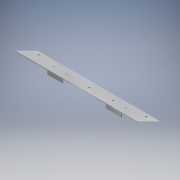
# Autodesk Inventor part: side plate
Saved by Autodesk Inventor 2016 (Build 200138000, 138)
## iProperties
Created: 2016-01-16
Part Number: side plate
Material: Aluminum 6061
Document SubType Name: Modeling
Designer: gus
Density: 2.7 g/cm^3
Appearance: Aluminum - Flat
Mass: 440.775 g
Surface Area: 1095.58 cm^2
Volume: 163.25 cm^3
User Status: complete
Author: gus
Autodesk Inventor part; units mm, degrees
ref_plane "YZ Plane" through (0, 0, 0) normal (1, 0, 0) x (0, 1, 0)
ref_plane "XZ Plane" through (0, 0, 0) normal (0, 1, 0) x (-1, 0, 0)
ref_plane "XY Plane" through (0, 0, 0) normal (0, 0, 1) x (1, 0, 0)
sketch "Sketch1" plane through (0, 0, 0) normal (0, 1, 0) x (-1, 0, 0)
  line L0 (0, 0) -> (762, 0)
  line L1 (762, 0) -> (762, 50.8)
  line L2 (762, 50.8) -> (0, 50.8)
  line L3 (0, 50.8) -> (0, 0)
  dimension "d0" = 762
  dimension "d1" = 50.8
  constraints: 8 end point, 2 parallel, 1 horizontal, 1 perpendicular
  measures "d0" distance of L2.end L1.end
  measures "d1" distance of L1.end L0.end
extrude "Extrusion1" add sketch "Sketch1" along normal blind 3.175
sketch "Sketch2" plane through (0, 3.175, 0) normal (0, 1, 0) x (1, 0, 0)
  circle A0 centre (-381, -28.575) radius 4.7625
  line L0 (0, 0) -> (-762, 0) projected
  line L1 (0, -50.8) -> (0, 0) projected
  circle A1 centre (-114.3, -12.7) radius 4.7625
  line L2 (-762, -50.8) -> (0, -50.8) projected
  circle A2 centre (-647.7, -12.7) radius 4.7625
  line L3 (-647.7, 0) -> (-647.7, -50.8) construction
  line L4 (-762, -50.8) -> (0, -50.8) construction
  line L5 (-114.3, -50.8) -> (-114.3, 0) construction
  circle A3 centre (-558.8, -25.4) radius 3.3734
  line L6 (-762, 0) -> (-762, -50.8) projected
  circle A4 centre (-495.3, -25.4) radius 3.3734
  circle A5 centre (-203.2, -25.4) radius 3.3734
  circle A6 centre (-266.7, -25.4) radius 3.3734
  dimension "d4" = 9.525
  dimension "d5" = 28.575
  dimension "d6" = 381
  dimension "d9" = 9.525
  dimension "d10" = 38.1
  dimension "d12" = 9.525
  dimension "d13" = 38.1
  dimension "d31" = 266.7
  dimension "d32" = 266.7
  dimension "d33" = 6.7469
  dimension "d34" = 203.2
  dimension "d35" = 25.4
  dimension "d36" = 6.7469
  dimension "d37" = 25.4
  dimension "d38" = 266.7
  dimension "d39" = 6.7469
  dimension "d40" = 6.7469
  dimension "d41" = 25.4
  dimension "d42" = 25.4
  dimension "d43" = 203.2
  dimension "d44" = 266.7
  constraints: 7 centre point, 6 point on line, 4 end point, 1 perpendicular, 1 vertical
  measures "d4" diameter of A0
  measures "d5" distance from line of L0 A0.centre
  measures "d6" distance from line of A0.centre L1
  measures "d9" diameter of A1
  measures "d10" distance from line of L2 A1.centre
  measures "d12" diameter of A2
  measures "d13" distance from line of L2 A2.centre
  measures "d31" distance from line of L3 A0.centre
  measures "d32" distance from line of L5 A0.centre
  measures "d33" diameter of A3
  measures "d34" distance from line of A3.centre L6
  measures "d35" distance from line of L0 A3.centre
  measures "d36" diameter of A4
  measures "d37" distance from line of L0 A4.centre
  measures "d38" distance from line of L6 A4.centre
  measures "d39" diameter of A5
  measures "d40" diameter of A6
  measures "d41" distance from line of L0 A6.centre
  measures "d42" distance from line of L0 A5.centre
  measures "d43" distance from line of L1 A5.centre
  measures "d44" distance from line of L1 A6.centre
extrude "Extrusion2" cut sketch "Sketch2" against normal blind 3.175 contours A0 | A1 | A2 | A3 | A4 | A5 | A6
sketch "Sketch3" plane through (-762, 0, 50.8) normal (0, 0, 1) x (1, 0, 0)
  line L0 (762, 3.175) -> (0, 3.175) projected
  line L1 (762, 3.175) -> (0, 3.175)
  line L2 (0, 3.175) -> (0, -19.05)
  line L3 (0, -19.05) -> (762, -19.05)
  line L4 (762, -19.05) -> (762, 3.175)
  point P0 (762, 0)
  dimension "d15" = 762
  dimension "d16" = 22.225
  constraints: 8 end point, 2 parallel, 1 horizontal, 1 perpendicular
  measures "d15" distance of L3.end L2.end
  measures "d16" distance of L2.end L1.end
extrude "Extrusion3" add sketch "Sketch3" along normal blind 3.175
sketch "Sketch4" plane through (0, 0, 0) normal (0, 0, -1) x (-1, 0, 0)
  line L0 (0, 3.175) -> (762, 3.175)
  line L1 (762, 3.175) -> (762, -19.05)
  line L2 (762, -19.05) -> (0, -19.05)
  line L3 (0, -19.05) -> (0, 3.175)
  dimension "d19" = 762
  dimension "d20" = 22.225
  constraints: 8 end point, 2 parallel, 1 horizontal, 1 perpendicular
  measures "d19" distance of L1.end L2.end
  measures "d20" distance of L0.end L1.end
extrude "Extrusion4" add sketch "Sketch4" along normal blind 3.175
sketch "Sketch5" plane through (-762, 0, 53.975) normal (0, 0, 1) x (1, 0, 0)
  line L0 (762, -19.05) -> (0, -19.05) projected
  line L1 (0, 0) -> (762, 0) projected
  line L2 (730.25, -19.05) -> (565.15, -19.05)
  line L3 (565.15, -19.05) -> (565.15, 0)
  line L4 (565.15, 0) -> (730.25, 0)
  line L5 (730.25, 0) -> (730.25, -19.05)
  line L6 (762, -19.05) -> (762, 3.175) projected
  line L7 (488.95, -19.05) -> (273.05, -19.05)
  line L8 (273.05, -19.05) -> (273.05, 0)
  line L9 (273.05, 0) -> (488.95, 0)
  line L10 (488.95, 0) -> (488.95, -19.05)
  line L11 (31.75, -19.05) -> (196.85, -19.05)
  line L12 (196.85, -19.05) -> (196.85, 0)
  line L13 (196.85, 0) -> (31.75, 0)
  line L14 (31.75, 0) -> (31.75, -19.05)
  line L15 (0, 3.175) -> (0, -19.05) projected
  dimension "d23" = 165.1
  dimension "d24" = 31.75
  dimension "d25" = 215.9
  dimension "d26" = 76.2
  dimension "d27" = 165.1
  dimension "d28" = 31.75
  constraints: 24 end point, 6 parallel, 6 point on line, 3 horizontal, 3 perpendicular
  measures "d23" distance of L3.end L4.end
  measures "d24" distance between parallel lines of L6 L5
  measures "d25" distance of L8.end L9.end
  measures "d26" distance between parallel lines of L10 L3
  measures "d27" distance of L12.end L13.end
  measures "d28" distance between parallel lines of L15 L14
extrude "Extrusion5" cut sketch "Sketch5" against normal blind 57.15 contours L0 L3 L1 L5 | L0 L8 L1 L10 | L0 L14 L1 L12
body "Solid1"
